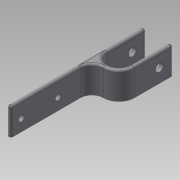
# Autodesk Inventor part: Ø12-Z Endstop Holder
Saved by Autodesk Inventor 2014 (Build 180170000, 170)
## iProperties
Created: 2015-08-05
Part Number: Ø12-Z Endstop Holder
Material: Generic
Document SubType Name: Modeling
Designer: Mathias L. Kjeldgaard
Density: 1 g/cm^3
Appearance: Default
Author: Mathias L. Kjeldgaard
Autodesk Inventor part; units mm, degrees
ref_plane "YZ Plane" through (0, 0, 0) normal (1, 0, 0) x (0, 1, 0)
ref_plane "XZ Plane" through (0, 0, 0) normal (0, 1, 0) x (-1, 0, 0)
ref_plane "XY Plane" through (0, 0, 0) normal (0, 0, 1) x (1, 0, 0)
sketch "Sketch1" plane through (0, 0, 0) normal (0, 0, 1) x (1, 0, 0)
  arc A0 (-6, 0) -> (6, 0) centre (0, 0) ccw
  arc A1 (0, -8) -> (8, 0) centre (0, 0) ccw
  line L0 (-6, -14) -> (-6, -50)
  line L1 (-8, 0) -> (-8, -50)
  line L2 (-6, 0) -> (-6, 20)
  line L3 (-8, 0) -> (-8, 20)
  line L4 (6, 0) -> (6, 20)
  line L5 (8, 0) -> (8, 20)
  line L6 (-8, -50) -> (-6, -50)
  line L7 (26.4346, -8) -> (-30.23, -8) construction
  arc A2 (0, -8) -> (-6, -14) centre (0, -14) ccw
  line L8 (8, 20) -> (6, 20)
  line L9 (-6, 20) -> (-8, 20)
  arc A3 (6, 0) -> (-6, 0) centre (0, 0) ccw construction
  dimension "d0" = 12
  dimension "d1" = 2
  dimension "d2" = 42
  dimension "d3" = 20
  dimension "d4" = 20
  constraints: 20 end point, 11 tangent, 8 point on circle, 7 parallel, 4 centre point, 2 coincident, 1 collinear, 1 perpendicular, 1 vertical
  measures "d0" diameter of A0
  measures "d1" radial gap between concentric circles of A1 A0
  measures "d2" distance between parallel lines of L6 L7
  measures "d3" distance from line of point (0, 0) L9
  measures "d4" distance from line of point (0, 0) L8
extrude "Extrusion1" add sketch "Sketch1" along normal blind 14
sketch "Sketch3" plane through (-8, -50, 0) normal (-1, 0, 0) x (0, 0, 1)
  line L0 (0, 0) -> (0, 70) projected
  line L1 (0, 0) -> (14, 0) projected
  line L2 (14, 70) -> (14, 0) projected
  line L3 (0, 70) -> (14, 70) projected
  line L4 (0, 42) -> (14, 42) projected
  circle A0 centre (6, 24.5) radius 1.5
  circle A1 centre (6, 5.5) radius 1.5
  line L5 (10.141, 23) -> (1.2635, 23) construction
  line L6 (10.6037, 7) -> (1.7262, 7) construction
  line L7 (6, 3.0673) -> (6, 29.9023) construction
  line L8 (9.9327, 26) -> (0.2455, 26) construction
  line L9 (10.6205, 4) -> (2.6453, 4) construction
  circle A2 centre (7, 63) radius 2
  line L10 (14, 54) -> (0, 54) construction
  point P0 (0, 50)
  dimension "d7" = 3
  dimension "d8" = 3
  dimension "d9" = 16
  dimension "d10" = 22
  dimension "d11" = 4
  dimension "d12" = 14
  dimension "d13" = 6
  dimension "d14" = 4
  dimension "d15" = 7
  dimension "d16" = 7
  dimension "d17" = 12
  constraints: 12 end point, 4 point on line, 4 tangent, 3 centre point, 3 parallel, 3 perpendicular
  measures "d7" diameter of A0
  measures "d8" diameter of A1
  measures "d9" distance between parallel lines of L5 L6
  measures "d10" distance between parallel lines of L8 L9
  measures "d11" distance between parallel lines of L1 L9
  measures "d12" distance between parallel lines of L2 L0
  measures "d13" distance between parallel lines of L0 L7
  measures "d14" diameter of A2
  measures "d15" distance from line of A2.centre L3
  measures "d16" distance from line of L2 A2.centre
  measures "d17" distance between parallel lines of L10 L4
extrude "Extrusion2" cut sketch "Sketch3" against normal up to surface (16 mm away) contours A0 | A1 | A2
fillet "Fillet1" radius 1 17 edges at (8, 20, 7) (6, 20, 7) (-6, 20, 7) (-8, 20, 7) (-6, -50, 7) (-8, -50, 7) (-4.2426, -9.7574, 14) (5.6569, -5.6569, 14) (8, 10, 14) (-6, -32, 14) (-6, 10, 14) (6, 10, 14) (0, -6, 14) (-8, -15, 14) (-7, -50, 14) (7, 20, 14) (-7, 20, 14)
equation "\"d4\" = d3"
equation "\"d8\" = d7"
equation "\"d16\" = 0.5 * d12"
body "Solid1"
